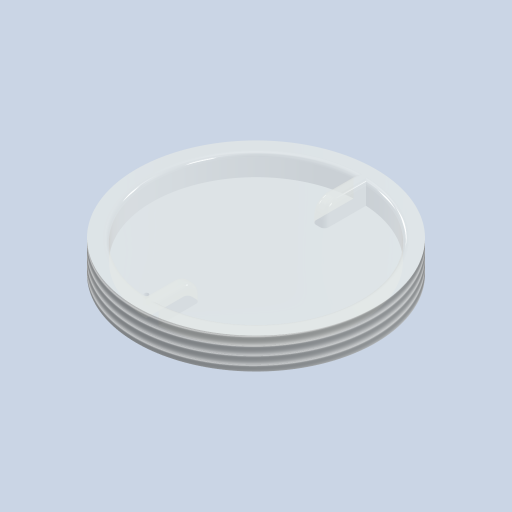
# Autodesk Inventor part: Capac
Saved by Autodesk Inventor 2024 (Build 280153000, 153)
## iProperties
Created: 2024-05-14
Part Number: Capac
Material: Glass
Document SubType Name: Modeling
Designer: mirun
Density: 2.18 g/cm^3
Appearance: Clear
Mass: 172.598 g
Surface Area: 297.353 cm^2
Volume: 79.1736 cm^3
Author: mirun
Autodesk Inventor part; units mm, degrees
ref_plane "YZ Plane" through (0, 0, 0) normal (1, 0, 0) x (0, 1, 0)
ref_plane "XZ Plane" through (0, 0, 0) normal (0, 1, 0) x (-1, 0, 0)
ref_plane "XY Plane" through (0, 0, 0) normal (0, 0, 1) x (1, 0, 0)
sketch "Sketch1" plane through (0, 0, 0) normal (0, 1, 0) x (-1, 0, 0)
  circle A0 centre (0, 0) radius 57.5
  dimension "d0" = 115
  constraints: 1 centre point, 1 coincident
  measures "d0" diameter of A0
extrude "Extrusion1" add sketch "Sketch1" along normal blind 15
sketch "Sketch2" plane through (0, 15, 0) normal (0, 1, 0) x (1, 0, 0)
  circle A0 centre (0, 0) radius 57.5 construction
  circle A1 centre (0, 0) radius 50
  dimension "d3" = 100
  constraints: 1 centre point, 1 coincident
  measures "d3" diameter of A1
extrude "Extrusion2" cut sketch "Sketch2" against normal blind 10
sketch "Sketch3" plane through (0, 5, 0) normal (0, 1, 0) x (1, 0, 0)
  circle A0 centre (0, 0) radius 50 construction
  line L0 (-3, -49.9099) -> (-3, -29.9099)
  line L1 (-3, -29.9099) -> (3, -29.9099)
  line L2 (3, -29.9099) -> (3, -49.9099)
  circle A1 centre (0, 0) radius 50
  line L3 (0, 0) -> (-15.0126, 0) construction
  circle A2 centre (0, 0) radius 50 construction
  line L4 (-3, 49.9099) -> (-3, 29.9099)
  line L5 (-3, 29.9099) -> (3, 29.9099)
  line L6 (3, 29.9099) -> (3, 49.9099)
  circle A3 centre (0, 0) radius 50
  dimension "d6" = 20
  dimension "d7" = 3
  dimension "d8" = 6
  constraints: 14 end point, 4 point on circle, 4 symmetric about line, 3 centre point, 2 coincident, 2 horizontal, 1 concentric, 1 perpendicular, 1 vertical, 2 other
  measures "d6" distance of L0.start L0.end
  measures "d7" distance from line of A0.centre L0
  measures "d8" distance of L0.end L1.end
extrude "Extrusion3" add sketch "Sketch3" along normal blind 10 contours L0 L1 L2 A1 | A1 L6 L5 L4
fillet "Fillet2" radius 7 2 edges at (0, 15, 29.9099) (0, 15, -29.9099)
fillet "Fillet3" radius 2 14 edges at (3, 12.9497, -31.9602) (3, 6.5, -29.9099) (3, 15, -43.4099) (-3, 12.9497, -31.9602) (-3, 6.5, -29.9099) (-3, 15, -43.4099) (-50, 15, 0) (50, 15, 0) (3, 12.9497, 31.9602) (3, 6.5, 29.9099) (3, 15, 43.4099) (-3, 12.9497, 31.9602) (-3, 6.5, 29.9099) (-3, 15, 43.4099)
thread "Thread1" size "M115x4" class "6g" standard "ANSI Metric M Profile" length 15
sketch "Sketch4" plane through (0, 5, 0) normal (0, 1, 0) x (1, 0, 0)
  circle A0 centre (-12.8327, -39.8572) radius 1
  dimension "d16" = 2
  constraints: 1 centre point
  measures "d16" diameter of A0
extrude "Extrusion4" cut sketch "Sketch4" against normal blind 10
body "Solid1"
